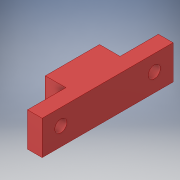
# Autodesk Inventor part: КВ33.044.202 - Фиксатор каретки
Saved by Autodesk Inventor 2019 (Build 230136000, 136)
## iProperties
Created: 2019-07-16
Part Number: КВ33.044.202 - Фиксатор каретки
Material: Пластик АБС
Document SubType Name: Modeling
Designer: Петров Иван
Density: 1.06 g/cm^3
Appearance: Гладкий — красный
Author: Петров Иван
Autodesk Inventor part; units mm, degrees
ref_plane "YZ Plane" through (0, 0, 0) normal (1, 0, 0) x (0, 1, 0)
ref_plane "XZ Plane" through (0, 0, 0) normal (0, 1, 0) x (-1, 0, 0)
ref_plane "XY Plane" through (0, 0, 0) normal (0, 0, 1) x (1, 0, 0)
sketch "Эскиз1" plane through (0, 0, 0) normal (1, 0, 0) x (0, 1, 0)
  line L0 (-9.5, 35) -> (9.5, 35)
  line L1 (9.5, 35) -> (9.5, -35)
  line L2 (9.5, -35) -> (-9.5, -35)
  line L3 (-9.5, -35) -> (-9.5, 35)
  line L4 (-9.5, 35) -> (9.5, -35) construction
  line L5 (9.5, 35) -> (-9.5, -35) construction
  line L6 (0, 35) -> (0, 25)
  circle A0 centre (0, 25) radius 3.25
  line L7 (0, -35) -> (0, -25)
  circle A1 centre (0, -25) radius 3.25
  point P0 (0, 0)
  dimension "d0" = 19
  dimension "d1" = 70
  dimension "d2" = 10
  dimension "d3" = 6.5
  dimension "d4" = 10
  dimension "d5" = 6.5
  constraints: 16 end point, 4 midpoint, 2 centre point, 2 coincident, 2 parallel, 2 vertical, 1 horizontal, 1 perpendicular
  measures "d0" distance of L1.end L2.end
  measures "d1" distance of L0.end L1.end
  measures "d2" distance of L6.start L6.end
  measures "d3" diameter of A0
  measures "d4" distance of L7.start L7.end
  measures "d5" diameter of A1
extrude "Выдавливание1" add sketch "Эскиз1" along normal blind 7.8
sketch "Эскиз2" plane through (0, 0, 0) normal (-1, 0, 0) x (0, 0, 1)
  line L0 (-35, 9.5) -> (35, 9.5) projected
  line L1 (-14.5, -9.5) -> (14.5, -9.5)
  line L2 (14.5, -9.5) -> (14.5, 9.5)
  line L3 (14.5, 9.5) -> (-14.5, 9.5)
  line L4 (-14.5, 9.5) -> (-14.5, -9.5)
  line L5 (-14.5, -9.5) -> (14.5, 9.5) construction
  line L6 (14.5, -9.5) -> (-14.5, 9.5) construction
  point P0 (0, 0)
  dimension "d8" = 29
  constraints: 12 end point, 2 midpoint, 2 parallel, 1 horizontal, 1 perpendicular, 1 point on line
  measures "d8" distance of L3.end L2.end
extrude "Выдавливание2" add sketch "Эскиз2" along normal blind 11
move faces "Перенос1" translate (0, -0.25, 0) faces at (5.2, -9.5, -4.8333)
move faces "Перенос3" translate (0, -1, 0) faces at (5.2, 9.5, 4.8333)
equation "\"d4\" = d2"
equation "\"d5\" = d3"
